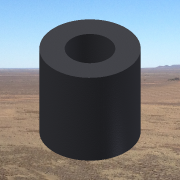
# Autodesk Inventor part: ductFan
Saved by Autodesk Inventor 2014 SP1 (Build 180222100, 222)
## iProperties
Created: 2014-05-22
Part Number: ductFan
Material: Iron, Ductile
Document SubType Name: Modeling
Designer: Dave
Mass: 87724.4 g
Surface Area: 5675.12 cm^2
Volume: 12355.6 cm^3
Density: 7.1 g/cm^3
Appearance: Iron - Cast
Author: Dave
Autodesk Inventor part; units mm, degrees
ref_plane "YZ Plane" through (0, 0, 0) normal (1, 0, 0) x (0, 1, 0)
ref_plane "XZ Plane" through (0, 0, 0) normal (0, 1, 0) x (-1, 0, 0)
ref_plane "XY Plane" through (0, 0, 0) normal (0, 0, 1) x (1, 0, 0)
sketch "Sketch1" plane through (0, 0, 0) normal (0, 1, 0) x (-1, 0, 0)
  circle A0 centre (0.5253, 0) radius 101.6
  circle A1 centre (0.5253, 0) radius 50.8
  point P0 (0, 0)
  dimension "d0" = 203.2
  dimension "d1" = 50.8
  constraints: 2 centre point
  measures "d0" diameter of A0
  measures "d1" radial gap between concentric circles of A1 A0
extrude "Extrusion1" add sketch "Sketch1" along normal blind 203.2
body "Solid1"
